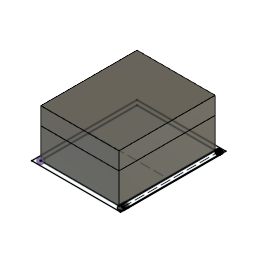
Stock Cutter (Autodesk Fusion 360 archive; units mm, degrees)
design "Stock Cutter"
part number: 1.625x2y-16
Autodesk Fusion 360 part; units mm, degrees
sketch "Stock" plane through (0, 0, 0) normal (0, 0, 1) x (1, 0, 0)
  line L0 (0, 0) -> (41.275, 0)
  line L1 (41.275, 0) -> (41.275, 50.8)
  line L2 (41.275, 50.8) -> (0, 50.8)
  line L3 (0, 50.8) -> (0, 0)
  line L4 (44.45, 1.7875) -> (44.45, 51)
  arc A0 (44.45, 51) -> (41.275, 51) centre (42.8625, 51) ccw
  line L5 (41.275, 51) -> (41.275, 1.7875)
  arc A1 (41.275, 1.7875) -> (44.45, 1.7875) centre (42.8625, 1.7875) ccw
  line L6 (42.8625, 0.2) -> (42.8625, 52.5875) construction
  line L7 (41.275, 51) -> (41.275, -0.2)
  arc A2 (41.275, -0.2) -> (44.45, -0.2) centre (42.8625, -0.2) ccw
  line L8 (44.45, -0.2) -> (44.45, 51)
  arc A3 (44.45, 51) -> (41.275, 51) centre (42.8625, 51) ccw
  line L9 (42.8625, 52.5875) -> (42.8625, -1.7875) construction
  line L10 (44.45, 53.1813) -> (-2.3813, 53.1813)
  line L11 (-2.3812, 53.1813) -> (-2.3813, -2.3813)
  line L12 (-2.3813, -2.3813) -> (44.45, -2.3813)
  line L13 (44.45, -2.3813) -> (44.45, 53.1813)
  line L14 (0, 25.4) -> (41.275, 25.4) construction
  dimension "d5" = 41.275
  dimension "d6" = 50.8
  dimension "d13" = 3.175
  dimension "d14" = 0.2
  dimension "d15" = 0.2
  dimension "d16" = 0.2
  dimension "d22" = 2.3813
  dimension "d23" = 2.3813
  constraint horizontal L0
  constraint vertical L1
  constraint horizontal L2
  constraint vertical L3
  constraint coincident L0.start L3.end
  constraint tangent L4 A0
  constraint tangent A0 L5
  constraint parallel L4 L5
  constraint tangent L5 A1
  constraint tangent L4 A1
  constraint midpoint A1 L6.start
  constraint midpoint A0 L6.end
  constraint vertical L6
  constraint collinear L1 L5
  constraint tangent L7 A2
  constraint tangent A2 L8
  constraint parallel L7 L8
  constraint tangent L8 A3
  constraint tangent L7 A3
  constraint midpoint A3 L6.end
  constraint midpoint A2 L9.end
  constraint vertical L9
  constraint equal A0 A3
  constraint coincident A0.centre A3.centre
  constraint horizontal L10
  constraint vertical L11
  constraint horizontal L12
  constraint vertical L13
  constraint coincident L8 L10.start
  constraint midpoint L3 L14.start
  constraint midpoint L7 L14.end
  constraint symmetric L10 L12 L14
  measures "d5" distance of L0.start L0.end
  measures "d6" distance of L0.start L2.end
  measures "d13" diameter of A0
  measures "d14" distance of L0 L6.start
  measures "d15" distance of L2 A0.centre
  measures "d16" distance of L0 A2.centre
  measures "d22" distance of L3 L11
  measures "d23" distance of L2 L10
extrude "Extrude1" add sketch "Stock" along normal blind 25.1714 contours L0 L1 L2 L3 L5 L7 makes body 1
ref_plane "WorkPlane1" through (20.6375, 25.4, 16) normal (0, 0, 1) x (1, 0, 0)
split "Split1" by plane through (20.6375, 25.4, 16) normal (0, 0, 1) bodies 1 makes body 2 at (13.7583, 17.5292, 25.1714)
equation "STOCK_Y = 2 in" comment "Desired stock dimensions"
equation "STOCK_X = 1.625 in"
equation "STOCK_Z = 0.991 in"
equation "ENDMILL_DIAMETER = 0.125 in"
equation "d5 = STOCK_X"
equation "d6 = STOCK_Y"
equation "d10 = STOCK_Z"
equation "d13 = ENDMILL_DIAMETER"
equation "CORNER_HEIGHT = 6 mm" comment "Height of the CNC mill corner"
equation "ENDMILL_LENGTH = 18 in" comment "Length of endmill cutter"
equation "CUT_DEPTH = min(ENDMILL_LENGTH; STOCK_Z / 2)" comment "Depth of the half slot we will cut"
equation "FACE_Z = 16 mm" comment "Height of top face when facing operation is selected"
equation "d21 = FACE_Z"
equation "d22 = ENDMILL_DIAMETER * 0.75"
equation "d23 = ENDMILL_DIAMETER * 0.75"
named bodies: "Base", "Top"
